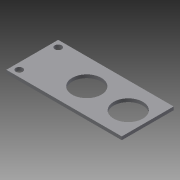
# Autodesk Inventor part: Bearing Plate 2-1
Saved by Autodesk Inventor 2013 (Build 170138000, 138)
## iProperties
Created: 2013-01-19
Part Number: Bearing Plate 2-1
Material: Generic
Document SubType Name: Modeling
Designer: actoennies
Density: 1 g/cm^3
Author: actoennies
Autodesk Inventor part; units mm, degrees
ref_plane "YZ Plane" through (0, 0, 0) normal (1, 0, 0) x (0, 1, 0)
ref_plane "XZ Plane" through (0, 0, 0) normal (0, 1, 0) x (-1, 0, 0)
ref_plane "XY Plane" through (0, 0, 0) normal (0, 0, 1) x (1, 0, 0)
sketch "Sketch1" plane through (0, 0, 0) normal (0, 1, 0) x (-1, 0, 0)
  circle A0 centre (0, 0) radius 14.2875
  circle A1 centre (87.63, -19.05) radius 3.3782
  circle A2 centre (87.63, 19.05) radius 3.3782
  circle A3 centre (40.64, 0) radius 14.2875
  line L0 (-19.05, 25.4) -> (93.98, 25.4)
  line L1 (93.98, 25.4) -> (93.98, -25.4)
  line L2 (93.98, -25.4) -> (-19.05, -25.4)
  line L3 (-19.05, -25.4) -> (-19.05, 25.4)
  dimension "d0" = 28.575
  dimension "d1" = 6.7564
  dimension "d2" = 6.7564
  dimension "d3" = 19.05
  dimension "d4" = 19.05
  dimension "d5" = 0
  dimension "d6" = 87.63
  dimension "d8" = 28.575
  dimension "d9" = 40.64
  dimension "d10" = 6.35
  dimension "d11" = 6.35
  dimension "d12" = 6.35
  dimension "d13" = 19.05
  constraints: 8 end point, 4 centre point, 2 parallel, 1 coincident, 1 horizontal, 1 perpendicular
  measures "d0" diameter of A0
  measures "d1" diameter of A1
  measures "d2" diameter of A2
  measures "d3" vertical distance of A2.centre A0.centre
  measures "d4" vertical distance of point (0, 0) A1.centre
  measures "d5" horizontal distance of A2.centre A1.centre
  measures "d6" horizontal distance of point (0, 0) A1.centre
  measures "d8" diameter of A3
  measures "d9" distance of point (0, 0) A3.centre
  measures "d10" distance from line of L0 A2.centre
  measures "d11" distance from line of L1 A2.centre
  measures "d12" distance from line of L2 A1.centre
  measures "d13" distance from line of L3 point (0, 0)
extrude "Extrusion1" add sketch "Sketch1" along normal blind 3.175
body "Solid1"
